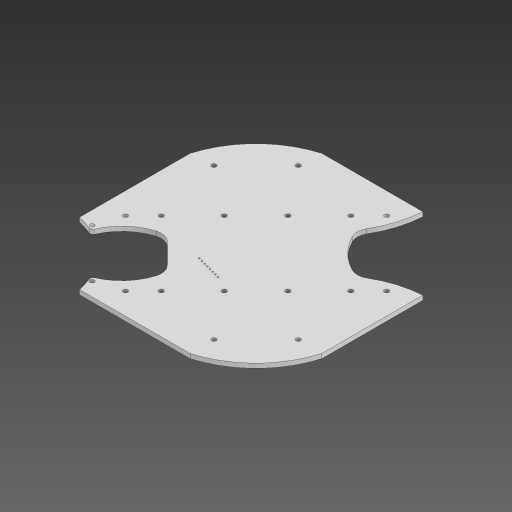
# Autodesk Inventor part: plata_v2
Saved by Autodesk Inventor 2023 (Build 270158000, 158)
## iProperties
Created: 2025-06-24
Part Number: plata_v2
Material: Типовые
Document SubType Name: Modeling
Designer: daa
Density: 1 g/cm^3
Appearance: По умолчанию
Author: daa
Autodesk Inventor part; units mm, degrees
ref_plane "YZ Plane" through (0, 0, 0) normal (1, 0, 0) x (0, 1, 0)
ref_plane "XZ Plane" through (0, 0, 0) normal (0, 1, 0) x (-1, 0, 0)
ref_plane "XY Plane" through (0, 0, 0) normal (0, 0, 1) x (1, 0, 0)
sketch "Эскиз1" plane through (0, 0, 0) normal (0, 1, 0) x (-1, 0, 0)
  line L0 (-79, -47.2724) -> (-79, 14.7276)
  line L1 (91.5447, -47.2724) -> (91.5447, 14.7276)
  line L2 (-79, -47.2724) -> (-93, -47.2724)
  line L3 (-79, 14.7276) -> (-93, 14.7276)
  line L4 (91.5447, -47.2724) -> (105.5447, -47.2724)
  line L5 (91.5447, 14.7276) -> (105.5447, 14.7276)
  line L6 (-24.7276, -101.5447) -> (37.2724, -101.5447)
  line L7 (-24.7276, 69) -> (37.2724, 69)
  line L8 (-24.7276, 69) -> (-24.7276, 83)
  line L9 (37.2724, 69) -> (37.2724, 83)
  line L10 (37.2724, -101.5447) -> (37.2724, -115.5447)
  line L11 (-24.7276, -101.5447) -> (-24.7276, -115.5447)
  arc A0 (-93, -47.2724) -> (-24.7276, -115.5447) centre (6.2724, -16.2724) ccw
  arc A1 (105.5447, 14.7276) -> (37.2724, 83) centre (6.2724, -16.2724) ccw
  arc A2 (-24.7276, 83) -> (-93, 14.7276) centre (6.2724, -16.2724) ccw
  arc A3 (37.2724, -115.5447) -> (105.5447, -47.2724) centre (6.2724, -16.2724) ccw
  dimension "d29" = 62
  dimension "d31" = 62
  dimension "d33" = 14
  dimension "d34" = 14
  dimension "d35" = 62
  dimension "d36" = 62
  dimension "d39" = 14
  dimension "d40" = 14
  constraints: 24 end point, 8 point on circle, 4 centre point, 4 horizontal, 3 parallel, 3 vertical, 2 point on line, 1 concentric
  measures "d29" distance of L0.start L0.end
  measures "d31" distance of L1.start L1.end
  measures "d33" distance of L0.end L3.end
  measures "d34" distance of L1.end L5.end
  measures "d35" distance of L6.start L6.end
  measures "d36" distance of L7.start L7.end
  measures "d39" distance of L7.start L8.end
  measures "d40" distance of L6.start L11.end
extrude "motor" add sketch "Эскиз1" along normal blind 3
sketch "Эскиз2" plane through (0, 3, 0) normal (0, 1, 0) x (1, 0, 0)
  arc A0 (24.7276, -83) -> (93, -14.7276) centre (-6.2724, 16.2724) ccw projected
  arc A1 (-37.2724, 115.5447) -> (-105.5447, 47.2724) centre (-6.2724, 16.2724) ccw projected
  circle A2 centre (-6.2724, 16.2724) radius 104
  line L0 (-6.2724, 16.2724) -> (-6.2724, -50.7276)
  arc A3 (-37.2724, 115.5447) -> (-105.5447, 47.2724) centre (-6.2724, 16.2724) ccw projected
  line L1 (-88.7917, -14.3063) -> (-40.8426, -62.2554)
  line L2 (-101.3809, -25.8032) -> (-48.3479, -78.8362)
  arc A4 (-105.5447, -14.7276) -> (-37.2724, -83) centre (-6.2724, 16.2724) ccw projected
  arc A5 (-48.3479, -78.8362) -> (-101.3809, -25.8032) centre (-98.035, -75.4903) ccw
  arc A6 (24.7276, -83) -> (93, -14.7276) centre (-6.2724, 16.2724) ccw projected
  line L3 (18.2427, 88.7365) -> (66.1918, 40.7874)
  line L4 (34.7276, 111.8495) -> (89.3048, 57.2724)
  arc A7 (34.7276, 111.8495) -> (89.3048, 57.2724) centre (70.9224, 93.4671) ccw
  line L5 (-91.5447, -14.7276) -> (-105.5447, -14.7276) projected
  arc A8 (-105.5447, -14.7276) -> (-101.3809, -25.8032) centre (-6.2724, 16.2724) ccw
  line L6 (-105.5447, -14.7276) -> (-80, -14.7276)
  line L7 (24.7276, 115.5447) -> (24.7276, 101.5447) projected
  line L8 (79, 47.2724) -> (93, 47.2724) projected
  arc A9 (89.3048, 57.2724) -> (34.7276, 111.8495) centre (-6.2724, 16.2724) ccw
  line L9 (93, 47.2724) -> (79, 47.2724)
  line L10 (24.7276, 115.5447) -> (24.7276, 101.5447)
  arc A10 (89.3048, 57.2724) -> (93, 47.2724) centre (-6.2724, 16.2724) ccw
  arc A11 (93, 47.2724) -> (24.7276, 115.5447) centre (-6.2724, 16.2724) ccw projected
  arc A12 (24.7276, 115.5447) -> (34.7276, 111.8495) centre (-6.2724, 16.2724) ccw
  line L11 (79, 47.2724) -> (59.7069, 47.2724)
  line L12 (24.7276, 101.5447) -> (24.7276, 82.2516)
  point P0 (0, 0)
  point P1 (-6.2724, -50.7276)
  point P2 (35.8032, 111.3809)
  point P3 (89.3048, 57.2724)
  point P4 (42.2173, 64.762)
  dimension "d181" = 208
  dimension "d190" = 67
  dimension "d205" = 75
  dimension "d207" = 17.0315
  dimension "d208" = 11.0756
  dimension "d209" = 104
  dimension "d316" = 28
  dimension "d317" = 10
  dimension "d318" = 10
  dimension "d330" = 40.5953
  constraints: 20 end point, 14 point on circle, 7 centre point, 4 point on line, 2 collinear, 2 tangent, 1 horizontal, 1 midpoint, 1 vertical
  measures "d181" diameter of A2
  measures "d190" distance of L0.end L0.start
  measures "d205" distance of L2.start L2.end
  measures "d207" distance between parallel lines of L1 L2
  measures "d208" horizontal distance of A2.end L2.end
  measures "d209" radius of A8
  measures "d316" distance from line of point (42.217, 64.762) L4
  measures "d317" distance from line of L7 L4.start
  measures "d318" distance from line of L4.end L8
  measures "d330" radius of A7
extrude "ball" cut sketch "Эскиз2" against normal blind 3 contours A2 L2 | L2 A5 | L4 A2 | A7 L4
sketch "Эскиз3" plane through (0, 3, 0) normal (0, 1, 0) x (1, 0, 0)
  arc A0 (93, 47.2724) -> (24.7276, 115.5447) centre (-6.2724, 16.2724) ccw projected
  line L0 (-6.2724, 16.2724) -> (97.7276, 16.2724) construction
  line L1 (67.2668, 89.8115) -> (-62.5447, -40)
  circle A1 centre (70.5306, -44.2673) radius 1.5
  circle A2 centre (54.2672, -60.5308) radius 1.5
  circle A3 centre (41.3053, -71.6104) radius 1.5
  circle A4 centre (81.6104, -31.3053) radius 1.5
  arc A5 (24.7276, -83) -> (93, -14.7276) centre (-6.2724, 16.2724) ccw projected
  line L2 (-6.2724, 16.2724) -> (97.7276, 16.2724) construction
  line L3 (-79.8115, 89.8115) -> (67.2668, -57.2668)
  line L4 (-91.5447, 47.2724) -> (-91.5447, -14.7276) projected
  line L5 (-91.5447, 16.2724) -> (79, 16.2724)
  line L6 (24.7276, 101.5447) -> (-37.2724, 101.5447) projected
  line L7 (-6.2724, 101.5447) -> (-6.2724, -69)
  line L8 (-6.2724, 101.5447) -> (-6.2724, -69)
  line L9 (-91.5447, 47.2724) -> (-91.5447, -14.7276) projected
  arc A6 (24.7276, -83) -> (93, -14.7276) centre (-6.2724, 16.2724) ccw projected
  circle A7 centre (-66.812, 93.0753) radius 1.5
  circle A8 centre (-83.0755, 76.8119) radius 1.5
  circle A9 centre (-94.1551, 63.85) radius 1.5
  circle A10 centre (-53.85, 104.1551) radius 1.5
  point P0 (0, 0)
  point P1 (67.2668, -57.2668)
  point P2 (67.2668, -57.2668)
  point P3 (-105.5447, 47.2724)
  point P4 (-79.8115, 89.8115)
  point P5 (-79.8115, 89.8115)
  point P6 (-79.8115, 89.8115)
  dimension "d65" = 3
  dimension "d66" = 3
  dimension "d67" = 3
  dimension "d68" = 3
  dimension "d69" = 23
  dimension "d71" = 57
  dimension "d74" = -12.962
  dimension "d78" = 25.9614
  constraints: 14 end point, 8 centre point, 8 symmetric about line, 4 point on circle, 3 midpoint, 2 horizontal, 2 vertical, 1 point on line, 4 other
  measures "d65" diameter of A1
  measures "d66" diameter of A2
  measures "d67" diameter of A3
  measures "d68" diameter of A4
  measures "d69" distance of A2.centre A1.centre
  measures "d71" distance of A3.centre A4.centre
  measures "d74" vertical distance of A1.centre A4.centre
  measures "d78" vertical distance of A4.centre point (67.267, -57.267)
extrude "hand_mount" cut sketch "Эскиз3" against normal blind 10
sketch "Эскиз5" plane through (0, 3, 0) normal (0, 1, 0) x (1, 0, 0)
  circle A0 centre (29.7645, -47.992) radius 1.5
  circle A1 centre (58.0485, -19.7074) radius 1.5
  circle A2 centre (-6.2982, 16.355) radius 104
  arc A3 (-105.5447, -14.7276) -> (-99.04, -30.7083) centre (-6.2982, 16.355) ccw projected
  line L0 (-6.2982, 16.355) -> (97.7018, 16.355) construction
  circle A4 centre (-71.4195, 53.192) radius 1.5
  circle A5 centre (-43.1349, 81.476) radius 1.5
  circle A6 centre (-45.0925, -54.9329) radius 1.5
  line L1 (-62.8214, -40.2767) -> (-61.356, -38.6694)
  line L2 (-61.356, -38.6694) -> (-45.4214, -38.6694) construction
  circle A7 centre (-77.6194, -22.406) radius 1.5
  arc A8 (24.7276, -83) -> (93, -14.7276) centre (-6.2724, 16.2724) ccw projected
  line L3 (-6.2982, 16.355) -> (97.7785, 16.355) construction
  line L4 (64.1086, -60.2947) -> (-82.2655, 87.2726)
  arc A9 (-37.2724, 115.5447) -> (-105.5447, 47.2724) centre (-6.2724, 16.2724) ccw projected
  circle A10 centre (27.3717, 81.7363) radius 1.5
  arc A11 (-48.3479, -78.8362) -> (-101.3809, -25.8032) centre (-98.035, -75.4903) ccw projected
  arc A12 (34.7276, 111.8495) -> (89.3048, 57.2724) centre (70.9224, 93.4671) ccw projected
  circle A13 centre (59.1841, 49.909) radius 1.5
  line L5 (27.3717, 81.7363) -> (71.0459, 81.7363) construction
  line L6 (27.3717, 81.7363) -> (59.1841, 49.909)
  line L7 (42.2173, 64.762) -> (43.2779, 65.8226)
  line L8 (42.2173, 64.762) -> (43.7173, 64.762) construction
  line L9 (-77.6194, -22.406) -> (-45.0925, -54.9329)
  line L10 (-77.6194, -22.406) -> (-31.6194, -22.406) construction
  point P0 (0, 0)
  point P1 (-62.8214, -40.2767)
  dimension "d116" = 3
  dimension "d117" = 3
  dimension "d118" = 40
  dimension "d119" = 208
  dimension "d121" = 64.347
  dimension "d126" = 3
  dimension "d130" = 2.175
  dimension "d332" = 45
  dimension "d335" = 1.5
  dimension "d336" = 45
  dimension "d337" = 46
  dimension "d338" = 45
  constraints: 22 end point, 9 centre point, 6 horizontal, 5 point on circle, 2 equal length, 2 midpoint, 1 coincident, 1 concentric, 1 symmetric about line, 1 other
  measures "d116" diameter of A0
  measures "d117" diameter of A1
  measures "d118" distance of A1.centre A0.centre
  measures "d119" diameter of A2
  measures "d121" vertical distance of L0.start A0.centre
  measures "d126" diameter of A6
  measures "d130" distance of L1.end L1.start
  measures "d332" distance of L5.start L6.end
  measures "d335" distance of L7.end L7.start
  measures "d336" angle of L8 L7
  measures "d337" distance of L9.start L9.end
  measures "d338" angle of L9 L10
extrude "Выдавливание5" cut sketch "Эскиз5" against normal blind 10 contours A0 | A1 | A4 | A5 | A6 | A7 | A10 | A13
sketch "Эскиз9" plane through (0, 3, 0) normal (0, 1, 0) x (1, 0, 0)
  line L0 (-38.87, 27.5154) -> (-17.5154, 48.87)
  line L1 (-17.5154, 48.87) -> (26.3253, 5.0294)
  line L2 (26.3253, 5.0294) -> (4.9706, -16.3253)
  line L3 (4.9706, -16.3253) -> (-38.87, 27.5154)
  circle A0 centre (-6.2724, 16.2724) radius 104
  arc A1 (-37.2724, 115.5447) -> (-105.5447, 47.2724) centre (-6.2724, 16.2724) ccw projected
  circle A2 centre (-17.5154, 48.87) radius 1.5
  circle A3 centre (-38.87, 27.5154) radius 1.5
  circle A4 centre (4.9706, -16.3253) radius 1.5
  circle A5 centre (26.3253, 5.0294) radius 1.5
  point P0 (0, 0)
  point P1 (-39.9194, 114.679)
  point P2 (-104.679, 49.9194)
  dimension "d224" = 30.2
  dimension "d225" = 62
  dimension "d226" = 208
  dimension "d227" = 15.1
  dimension "d229" = 31
  dimension "d230" = 3
  dimension "d231" = 3
  dimension "d232" = 3
  dimension "d233" = 3
  constraints: 8 end point, 5 centre point, 4 coincident, 2 parallel, 1 concentric, 1 perpendicular
  measures "d224" distance of L1.end L2.end
  measures "d225" distance of L0.end L1.end
  measures "d226" diameter of A0
  measures "d227" distance from line of L1 A0.centre
  measures "d229" distance from line of L2 A0.centre
  measures "d230" diameter of A2
  measures "d231" diameter of A3
  measures "d232" diameter of A4
  measures "d233" diameter of A5
extrude "Выдавливание8" cut sketch "Эскиз9" against normal blind 10 contours L3 A3 L0 | L0 A3 L3 | A2 L1 L0 | L0 L1 A2 | A4 L2 L3 | L3 L2 A4 | A5 L2 L1 | L1 L2 A5
sketch "Эскиз8" plane through (0, 3, 0) normal (0, 1, 0) x (1, 0, 0)
  circle A0 centre (62.3989, -52.3991) radius 1.6
  circle A1 centre (54.2672, -60.5308) radius 1.5
  circle A2 centre (54.2672, -60.5308) radius 1.5 projected
  line L0 (54.2672, -60.5308) -> (67.7672, -60.5308) construction
  circle A3 centre (70.5306, -44.2673) radius 1.5
  circle A4 centre (70.5306, -44.2673) radius 1.5 projected
  line L1 (70.5306, -44.2673) -> (82.0306, -44.2673) construction
  line L2 (70.5306, -44.2673) -> (60.52, -44.2673)
  circle A5 centre (70.5306, -44.2673) radius 1.5 projected
  line L3 (60.52, -44.2673) -> (70.5306, -44.2673)
  line L4 (70.5306, -44.2673) -> (62.3989, -52.3991)
  arc A6 (34.7276, 111.8495) -> (89.3048, 57.2724) centre (70.9224, 93.4671) ccw projected
  arc A7 (93, 47.2724) -> (89.3048, 57.2724) centre (-6.2724, 16.2724) ccw projected
  line L5 (24.7276, 115.5447) -> (24.7276, 101.5447) projected
  line L6 (24.7276, 101.5447) -> (-37.2724, 101.5447) projected
  line L7 (-37.2724, 101.5447) -> (-37.2724, 115.5447) projected
  arc A8 (-37.2724, 115.5447) -> (-105.5447, 47.2724) centre (-6.2724, 16.2724) ccw projected
  line L8 (-105.5447, 47.2724) -> (-91.5447, 47.2724) projected
  line L9 (-91.5447, 47.2724) -> (-91.5447, -14.7276) projected
  line L10 (-91.5447, -14.7276) -> (-105.5447, -14.7276) projected
  arc A9 (-105.5447, -14.7276) -> (-101.3809, -25.8032) centre (-6.2724, 16.2724) ccw projected
  arc A10 (-48.3479, -78.8362) -> (-101.3809, -25.8032) centre (-98.035, -75.4903) ccw projected
  arc A11 (-48.3479, -78.8362) -> (-37.2724, -83) centre (-6.2724, 16.2724) ccw projected
  line L11 (-37.2724, -83) -> (-37.2724, -69) projected
  line L12 (-37.2724, -69) -> (24.7276, -69) projected
  line L13 (24.7276, -69) -> (24.7276, -83) projected
  arc A12 (24.7276, -83) -> (93, -14.7276) centre (-6.2724, 16.2724) ccw projected
  line L14 (93, -14.7276) -> (79, -14.7276) projected
  line L15 (79, -14.7276) -> (79, 47.2724) projected
  line L16 (79, 47.2724) -> (93, 47.2724) projected
  arc A13 (34.7276, 111.8495) -> (24.7276, 115.5447) centre (-6.2724, 16.2724) ccw projected
  circle A14 centre (-94.1551, 63.85) radius 1.5 projected
  circle A15 centre (41.3053, -71.6104) radius 1.5 projected
  circle A16 centre (81.6104, -31.3053) radius 1.5 projected
  circle A17 centre (-53.85, 104.1551) radius 1.5 projected
  circle A18 centre (-83.0755, 76.8119) radius 1.5 projected
  circle A19 centre (54.2672, -60.5308) radius 1.5 projected
  circle A20 centre (70.5306, -44.2673) radius 1.5 projected
  circle A21 centre (-66.812, 93.0753) radius 1.5 projected
  circle A22 centre (-45.0925, -54.9329) radius 1.5 projected
  circle A23 centre (29.7645, -47.992) radius 1.5 projected
  circle A24 centre (-43.1349, 81.476) radius 1.5 projected
  circle A25 centre (27.3717, 81.7363) radius 1.5 projected
  circle A26 centre (-77.6194, -22.406) radius 1.5 projected
  circle A27 centre (58.0485, -19.7074) radius 1.5 projected
  circle A28 centre (-71.4195, 53.192) radius 1.5 projected
  line L17 (42.2173, 64.762) -> (-62.8214, -40.2767)
  arc A29 (-48.275, -77.4757) -> (-100.0204, -25.7303) centre (-98.035, -75.4903) ccw projected
  circle A30 centre (-74.9438, 84.9436) radius 1.6
  point P0 (0, 0)
  dimension "d212" = 3.2
  dimension "d216" = 3
  dimension "d221" = 3
  dimension "d311" = 11.5
  dimension "d312" = 45
  constraints: 12 end point, 4 centre point, 3 horizontal, 3 point on circle, 2 concentric, 1 coincident, 1 collinear, 1 symmetric about line, 1 other
  measures "d212" diameter of A0
  measures "d216" diameter of A1
  measures "d221" diameter of A3
  measures "d311" distance of L3.end L4.end
  measures "d312" angle of L3 L4
extrude "Выдавливание7" cut sketch "Эскиз8" against normal blind 10 contours A0 | A30
sketch "Эскиз10" plane through (0, 3, 0) normal (0, 1, 0) x (1, 0, 0)
  circle A0 centre (-6.2724, 16.2719) radius 104.0005
  arc A1 (-37.2724, 115.5447) -> (-105.5447, 47.2724) centre (-6.2724, 16.2724) ccw projected
  line L0 (-60.0125, 6.3729) -> (-72.0333, -5.648)
  line L1 (-72.0333, -5.648) -> (-28.1927, -49.4886)
  line L2 (-28.1927, -49.4886) -> (-16.1718, -37.4678)
  line L3 (-16.1718, -37.4678) -> (-60.0125, 6.3729)
  circle A2 centre (-60.0125, 6.3729) radius 1.5
  circle A3 centre (-72.0333, -5.648) radius 1.5
  circle A4 centre (-16.1718, -37.4678) radius 1.5
  circle A5 centre (-28.1927, -49.4886) radius 1.5
  arc A6 (24.7276, -83) -> (93, -14.7276) centre (-6.2724, 16.2724) ccw projected
  line L4 (-6.2724, 16.2724) -> (97.7276, 16.2724) construction
  line L5 (67.2668, -57.2668) -> (-79.8115, 89.8115)
  line L6 (3.6271, 70.0125) -> (15.648, 82.0333)
  line L7 (15.648, 82.0333) -> (59.4886, 38.1927)
  line L8 (59.4886, 38.1927) -> (47.4678, 26.1718)
  line L9 (47.4678, 26.1718) -> (3.6271, 70.0125)
  circle A7 centre (3.6271, 70.0125) radius 1.5
  circle A8 centre (15.648, 82.0333) radius 1.5
  circle A9 centre (47.4678, 26.1718) radius 1.5
  circle A10 centre (59.4886, 38.1927) radius 1.5
  point P0 (0, 0)
  point P1 (-39.9194, 114.679)
  point P2 (-104.679, 49.9194)
  point P3 (27.3747, -82.1343)
  point P4 (92.1343, -17.3747)
  point P5 (10, 10)
  point P6 (-6.2719, 16.2724)
  dimension "d248" = 17
  dimension "d249" = 62
  dimension "d250" = 9.899
  dimension "d251" = 45
  dimension "d252" = 3
  dimension "d253" = 3
  dimension "d254" = 3
  dimension "d255" = 3
  constraints: 20 end point, 10 symmetric about line, 9 centre point, 8 coincident, 2 parallel, 2 point on circle, 1 horizontal, 1 perpendicular, 1 tangent, 4 other
  measures "d248" distance of L2.end L1.end
  measures "d249" distance of L1.end L0.end
  measures "d250" vertical distance of L0.start A0.centre
  measures "d251" distance from line of L3 L4.start
  measures "d252" diameter of A2
  measures "d253" diameter of A3
  measures "d254" diameter of A4
  measures "d255" diameter of A5
extrude "Выдавливание9" cut sketch "Эскиз10" against normal blind 10 contours L3 A2 L0 | L0 A2 L3 | A3 L1 L0 | L0 L1 A3 | A4 L2 L3 | L3 L2 A4 | A5 L2 L1 | L1 L2 A5 | L9 A7 L6 | L6 A7 L9 | A8 L7 L6 | L6 L7 A8 | A9 L8 L9 | L9 L8 A9 | A10 L8 L7 | L7 L8 A10
sketch "Эскиз19" plane through (0, 3, 0) normal (0, 1, 0) x (1, 0, 0)
  circle A0 centre (47.4678, 26.1718) radius 1.5 projected
  circle A1 centre (-28.1927, -49.4886) radius 1.5 projected
  circle A2 centre (-72.0333, -5.648) radius 1.5 projected
  circle A3 centre (15.648, 82.0333) radius 1.5 projected
  circle A4 centre (59.4886, 38.1927) radius 1.5 projected
  circle A5 centre (-16.1718, -37.4678) radius 1.5 projected
  circle A6 centre (-60.0125, 6.3729) radius 1.5 projected
  circle A7 centre (3.6271, 70.0125) radius 1.5 projected
  circle A8 centre (4.9706, -16.3253) radius 1.5 projected
  circle A9 centre (-17.5154, 48.87) radius 1.5 projected
  circle A10 centre (26.3253, 5.0294) radius 1.5 projected
  circle A11 centre (-38.87, 27.5154) radius 1.5 projected
  circle A12 centre (62.3989, -52.3991) radius 1.6 projected
  circle A13 centre (-74.9438, 84.9436) radius 1.6 projected
  circle A14 centre (58.0485, -19.7074) radius 1.5 projected
  circle A15 centre (-71.4195, 53.192) radius 1.5 projected
  circle A16 centre (27.3717, 81.7363) radius 1.5 projected
  circle A17 centre (-77.6194, -22.406) radius 1.5 projected
  circle A18 centre (29.7645, -47.992) radius 1.5 projected
  circle A19 centre (-43.1349, 81.476) radius 1.5 projected
  circle A20 centre (59.1841, 49.909) radius 1.5 projected
  circle A21 centre (-45.0925, -54.9329) radius 1.5 projected
  circle A22 centre (-66.812, 93.0753) radius 1.5 projected
  circle A23 centre (70.5306, -44.2673) radius 1.5 projected
  circle A24 centre (54.2672, -60.5308) radius 1.5 projected
  circle A25 centre (-83.0755, 76.8119) radius 1.5 projected
  circle A26 centre (-53.85, 104.1551) radius 1.5 projected
  circle A27 centre (81.6104, -31.3053) radius 1.5 projected
  circle A28 centre (41.3053, -71.6104) radius 1.5 projected
  circle A29 centre (-94.1551, 63.85) radius 1.5 projected
  arc A30 (34.7276, 111.8495) -> (89.3048, 57.2724) centre (70.9224, 93.4671) ccw projected
  arc A31 (34.7276, 111.8495) -> (24.7276, 115.5447) centre (-6.2724, 16.2724) ccw projected
  line L0 (24.7276, 115.5447) -> (24.7276, 101.5447) projected
  line L1 (24.7276, 101.5447) -> (-37.2724, 101.5447) projected
  line L2 (-37.2724, 101.5447) -> (-37.2724, 115.5447) projected
  arc A32 (-37.2724, 115.5447) -> (-105.5447, 47.2724) centre (-6.2724, 16.2724) ccw projected
  line L3 (-105.5447, 47.2724) -> (-91.5447, 47.2724) projected
  line L4 (-91.5447, 47.2724) -> (-91.5447, -14.7276) projected
  line L5 (-91.5447, -14.7276) -> (-105.5447, -14.7276) projected
  arc A33 (-105.5447, -14.7276) -> (-101.3809, -25.8032) centre (-6.2724, 16.2724) ccw projected
  arc A34 (-48.3479, -78.8362) -> (-101.3809, -25.8032) centre (-98.035, -75.4903) ccw projected
  arc A35 (-48.3479, -78.8362) -> (-37.2724, -83) centre (-6.2724, 16.2724) ccw projected
  line L6 (-37.2724, -83) -> (-37.2724, -69) projected
  line L7 (-37.2724, -69) -> (24.7276, -69) projected
  line L8 (24.7276, -69) -> (24.7276, -83) projected
  arc A36 (24.7276, -83) -> (93, -14.7276) centre (-6.2724, 16.2724) ccw projected
  line L9 (93, -14.7276) -> (79, -14.7276) projected
  line L10 (79, -14.7276) -> (79, 47.2724) projected
  line L11 (79, 47.2724) -> (93, 47.2724) projected
  arc A37 (93, 47.2724) -> (89.3048, 57.2724) centre (-6.2724, 16.2724) ccw projected
  arc A38 (-42.2724, 108.4949) -> (-98.4949, 52.2724) centre (-6.2724, 16.2724) ccw
  line L12 (-42.2724, 108.4949) -> (-42.2724, 96.5447)
  line L13 (-42.2724, 96.5447) -> (25.4312, 96.5447)
  arc A39 (25.4312, 96.5447) -> (74, 47.9759) centre (70.9224, 93.4671) ccw
  line L14 (74, 47.9759) -> (74, -19.7276)
  line L15 (74, -19.7276) -> (85.9502, -19.7276)
  arc A40 (29.7276, -75.9502) -> (85.9502, -19.7276) centre (-6.2724, 16.2724) ccw
  line L16 (29.7276, -75.9502) -> (29.7276, -64)
  line L17 (-86.5447, 52.2724) -> (-98.4949, 52.2724)
  arc A41 (-42.2724, 96.5447) -> (-86.5447, 52.2724) centre (-24.1284, 34.1284) ccw
  arc A42 (29.7276, -64) -> (74, -19.7276) centre (11.5837, -1.5837) ccw
  line L18 (-86.5447, 52.2724) -> (-86.5447, -21.9089)
  line L19 (29.7276, -64) -> (-44.4536, -64)
  arc A43 (-44.4536, -64) -> (-86.5447, -21.9089) centre (-98.035, -75.4903) ccw
  point P0 (0, 0)
  point P1 (26.5474, 82.9894)
  point P2 (27.2884, 80.2386)
  point P3 (57.6859, 49.8355)
  point P4 (60.4425, 49.0926)
  dimension "d339" = 5
  dimension "d340" = 65
  dimension "d341" = 65
  constraints: 16 end point, 12 point on circle, 6 centre point, 1 perpendicular, 1 vertical, 7 other
  measures "d339" radial gap between concentric circles of A32 A38
  measures "d340" radius of A41
  measures "d341" radius of A42
extrude "Выдавливание13" cut sketch "Эскиз19" against normal blind 10 contours A41 L17 A38 A29 A25 A22 A26 L12 | L15 A40 A27 A23 A24 A28 L16 A42 | A30 A37 L11 L10 L9 A36 L8 L7 L6 A35 A34 A33 L5 L4 L3 A32 L2 L1 L0 A31
sketch "Эскиз20" plane through (0, 3, 0) normal (0, 1, 0) x (1, 0, 0)
  circle A0 centre (-45.0925, -54.9329) radius 1.5 projected
  circle A1 centre (-43.1349, 81.476) radius 1.5 projected
  circle A2 centre (29.7645, -47.992) radius 1.5 projected
  circle A3 centre (-77.6194, -22.406) radius 1.5 projected
  circle A4 centre (-71.4195, 53.192) radius 1.5 projected
  circle A5 centre (58.0485, -19.7074) radius 1.5 projected
  circle A6 centre (-38.87, 27.5154) radius 1.5 projected
  circle A7 centre (26.3253, 5.0294) radius 1.5 projected
  circle A8 centre (-17.5154, 48.87) radius 1.5 projected
  circle A9 centre (4.9706, -16.3253) radius 1.5 projected
  circle A10 centre (3.6271, 70.0125) radius 1.5 projected
  circle A11 centre (-60.0125, 6.3729) radius 1.5 projected
  circle A12 centre (-16.1718, -37.4678) radius 1.5 projected
  circle A13 centre (59.4886, 38.1927) radius 1.5 projected
  circle A14 centre (15.648, 82.0333) radius 1.5 projected
  circle A15 centre (-72.0333, -5.648) radius 1.5 projected
  circle A16 centre (-28.1927, -49.4886) radius 1.5 projected
  circle A17 centre (47.4678, 26.1718) radius 1.5 projected
  arc A18 (25.4312, 96.5447) -> (26.5474, 82.9894) centre (70.9224, 93.4671) ccw projected
  line L0 (25.4312, 96.5447) -> (-42.2724, 96.5447) projected
  arc A19 (-42.2724, 96.5447) -> (-86.5447, 52.2724) centre (-24.1284, 34.1284) ccw projected
  line L1 (-86.5447, 52.2724) -> (-86.5447, -21.9089) projected
  arc A20 (-44.4536, -64) -> (-86.5447, -21.9089) centre (-98.035, -75.4903) ccw projected
  line L2 (-44.4536, -64) -> (29.7276, -64) projected
  arc A21 (29.7276, -64) -> (74, -19.7276) centre (11.5837, -1.5837) ccw projected
  line L3 (74, -19.7276) -> (74, 47.9759) projected
  arc A22 (60.4425, 49.0926) -> (74, 47.9759) centre (70.9224, 93.4671) ccw projected
  arc A23 (57.6859, 49.8355) -> (60.4425, 49.0926) centre (59.1841, 49.909) ccw projected
  arc A24 (27.2884, 80.2386) -> (57.6859, 49.8355) centre (70.9224, 93.4671) ccw projected
  arc A25 (26.5474, 82.9894) -> (27.2884, 80.2386) centre (27.3717, 81.7363) ccw projected
  arc A26 (-44.4536, -64) -> (-86.5447, -21.9089) centre (-98.035, -75.4903) ccw projected
  line L4 (-71.3723, -27.6144) -> (-50.1591, -48.8276)
  line L5 (-50.1591, -48.8276) -> (-25.4104, -24.0789)
  line L6 (-25.4104, -24.0789) -> (-46.6236, -2.8657)
  line L7 (-46.6236, -2.8657) -> (-71.3723, -27.6144)
  arc A27 (-46.6236, -2.8657) -> (-75.3457, -25.6085) centre (-42.4708, -37.6184) ccw
  line L8 (-36.017, -13.4723) -> (-60.7657, -38.221)
  arc A28 (-48.1532, -52.801) -> (-25.4104, -24.0789) centre (-60.1632, -19.9261) ccw
  line L9 (-8.4206, 14.1241) -> (55.3471, -49.6436)
  arc A29 (29.7276, -64) -> (74, -19.7276) centre (11.5837, -1.5837) ccw projected
  line L10 (-8.4206, 14.1241) -> (81.7606, 14.1241) construction
  line L11 (55.3471, -49.6436) -> (-72.1883, 77.8919)
  arc A30 (-42.2724, 96.5447) -> (-86.5447, 52.2724) centre (-24.1284, 34.1284) ccw projected
  line L12 (28.0624, 77.9125) -> (55.3265, 50.6222)
  line L13 (55.3265, 50.6222) -> (41.1775, 36.4868)
  line L14 (41.1775, 36.4868) -> (13.9134, 63.7772)
  line L15 (13.9134, 63.7772) -> (28.0624, 77.9125)
  arc A31 (26.5474, 82.9894) -> (27.2884, 80.2386) centre (27.3717, 81.7363) ccw projected
  arc A32 (13.9134, 63.7772) -> (41.1775, 36.4868) centre (56.3081, 78.8669) ccw
  arc A33 (13.9134, 63.7772) -> (25.4312, 96.5447) centre (-39.4206, 100.932) ccw
  arc A34 (74, 47.9759) -> (41.1775, 36.4868) centre (78.2808, -16.883) ccw
  point P0 (0, 0)
  point P1 (-75.3457, -25.6085)
  point P2 (73.9122, 47.97)
  dimension "d357" = 35
  dimension "d363" = 35
  dimension "d368" = 45
  dimension "d369" = 20
  dimension "d372" = 45
  dimension "d382" = 65
  dimension "d383" = 65
  constraints: 24 end point, 17 point on circle, 5 centre point, 4 parallel, 2 midpoint, 2 perpendicular, 2 symmetric about line, 1 equal length, 1 horizontal, 1 point on line, 1 tangent, 1 other
  measures "d357" distance of L5.end L4.end
  measures "d363" radius of A27
  measures "d368" angle of L9 L10
  measures "d369" distance of L12.end L13.end
  measures "d372" radius of A32
  measures "d382" radius of A33
  measures "d383" radius of A34
extrude "Выдавливание14" cut sketch "Эскиз20" against normal blind 10 contours A18 A25 A24 L15 A33 | L15 A24 L13 L14 | L14 A32 | L13 A24 A23 A22 A34 | A27 L7 A20 | L7 L6 L8 A20 | L8 L6 L5 A20 | A20 L5 A28
fillet "Сопряжение12" radius 10 2 edges at (-46.6236, 1.5, 2.8657) (-25.4104, 1.5, 24.0789)
fillet "Сопряжение13" radius 2 2 edges at (-75.3457, 1.5, 25.6085) (-48.1532, 1.5, 52.801)
fillet "Сопряжение14" radius 10 2 edges at (13.9134, 1.5, -63.7772) (41.1775, 1.5, -36.4868)
sketch "Эскиз21" plane through (0, 3, 0) normal (0, 1, 0) x (1, 0, 0)
  circle A0 centre (9.8791, 38.23) radius 0.45 projected
  circle A1 centre (7.4254, 38.8877) radius 0.45 projected
  circle A2 centre (4.9725, 39.5446) radius 0.45 projected
  ellipse E0 centre (-6.272, 16.272) end of major axis (-21.0463, 59.1087) minor radius 45.313 projected
  circle A3 centre (-12.1713, -26.3968) radius 0.425 projected
  circle A4 centre (-17.1529, -25.4059) radius 0.425 projected
  circle A5 centre (-14.6618, -25.9017) radius 0.425 projected
  circle A6 centre (-3.7334, -26.7287) radius 0.425 projected
  circle A7 centre (-8.8133, -26.7285) radius 0.425 projected
  circle A8 centre (-6.2734, -26.7286) radius 0.425 projected
  circle A9 centre (-30.1627, -19.4807) radius 0.425 projected
  circle A10 centre (-34.8635, -15.9096) radius 0.425 projected
  circle A11 centre (-32.2833, -18.0827) radius 0.425 projected
  circle A12 centre (-22.7291, -23.4541) radius 0.425 projected
  circle A13 centre (-20.3822, -24.4265) radius 0.425 projected
  circle A14 centre (-28.0422, -20.8787) radius 0.425 projected
  circle A15 centre (-25.0752, -22.4825) radius 0.425 projected
  circle A16 centre (17.6165, -19.4822) radius 0.425 projected
  circle A17 centre (12.5287, -22.4837) radius 0.425 projected
  circle A18 centre (15.5043, -20.8928) radius 0.425 projected
  circle A19 centre (24.1326, -14.1346) radius 0.425 projected
  circle A20 centre (25.9287, -12.3386) radius 0.425 projected
  circle A21 centre (19.7279, -18.0709) radius 0.425 projected
  circle A22 centre (22.3365, -15.9306) radius 0.425 projected
  circle A23 centre (4.6062, -25.4066) radius 0.425 projected
  circle A24 centre (-0.3754, -26.3971) radius 0.425 projected
  circle A25 centre (2.1151, -25.9022) radius 0.425 projected
  circle A26 centre (7.8356, -24.4274) radius 0.425 projected
  circle A27 centre (10.1825, -23.4552) radius 0.425 projected
  ellipse E1 centre (4.9707, -16.3253) end of major axis (3.8747, -15.2292) minor radius 1.55 projected
  line L0 (19.1105, -0.9108) -> (18.6169, -1.4765) projected
  line L1 (18.6169, -1.4765) -> (11.4756, -8.6187) projected
  line L2 (11.4756, -8.6187) -> (10.9099, -9.1123) projected
  line L3 (10.9099, -9.1123) -> (10.282, -9.5238) projected
  line L4 (10.282, -9.5238) -> (9.6046, -9.8462) projected
  line L5 (9.6046, -9.8462) -> (8.8882, -10.0732) projected
  line L6 (8.8882, -10.0732) -> (8.1486, -10.2004) projected
  line L7 (8.1486, -10.2004) -> (7.3984, -10.2266) projected
  line L8 (7.3984, -10.2266) -> (6.6524, -10.1495) projected
  line L9 (6.6524, -10.1495) -> (5.9226, -9.9713) projected
  line L10 (5.9226, -9.9713) -> (5.2247, -9.6962) projected
  line L11 (5.2247, -9.6962) -> (4.57, -9.3285) projected
  line L12 (4.57, -9.3285) -> (3.9718, -8.8745) projected
  line L13 (3.9718, -8.8745) -> (3.4415, -8.3441) projected
  line L14 (3.4415, -8.3441) -> (2.9875, -7.7459) projected
  line L15 (2.9875, -7.7459) -> (2.6198, -7.0911) projected
  line L16 (2.6198, -7.0911) -> (2.3448, -6.3932) projected
  line L17 (2.3448, -6.3932) -> (2.1666, -5.6634) projected
  line L18 (2.1666, -5.6634) -> (2.0896, -4.9174) projected
  line L19 (2.0896, -4.9174) -> (2.1158, -4.1672) projected
  line L20 (2.1158, -4.1672) -> (2.2431, -3.4276) projected
  line L21 (2.2431, -3.4276) -> (2.4701, -2.7113) projected
  line L22 (2.4701, -2.7113) -> (2.7925, -2.0339) projected
  line L23 (2.7925, -2.0339) -> (3.2041, -1.406) projected
  line L24 (3.2041, -1.406) -> (3.6977, -0.8403) projected
  line L25 (3.6977, -0.8403) -> (10.839, 6.3019) projected
  line L26 (10.839, 6.3019) -> (11.4047, 6.7955) projected
  line L27 (11.4047, 6.7955) -> (12.0326, 7.207) projected
  line L28 (12.0326, 7.207) -> (12.71, 7.5294) projected
  line L29 (12.71, 7.5294) -> (13.4263, 7.7564) projected
  line L30 (13.4263, 7.7564) -> (14.166, 7.8836) projected
  line L31 (14.166, 7.8836) -> (14.9162, 7.9098) projected
  line L32 (14.9162, 7.9098) -> (15.6622, 7.8327) projected
  line L33 (15.6622, 7.8327) -> (16.3919, 7.6545) projected
  line L34 (16.3919, 7.6545) -> (17.0898, 7.3794) projected
  line L35 (17.0898, 7.3794) -> (17.7446, 7.0117) projected
  line L36 (17.7446, 7.0117) -> (18.3428, 6.5577) projected
  line L37 (18.3428, 6.5577) -> (18.8731, 6.0273) projected
  line L38 (18.8731, 6.0273) -> (19.3271, 5.4291) projected
  line L39 (19.3271, 5.4291) -> (19.6947, 4.7743) projected
  line L40 (19.6947, 4.7743) -> (19.9698, 4.0764) projected
  line L41 (19.9698, 4.0764) -> (20.1479, 3.3466) projected
  line L42 (20.1479, 3.3466) -> (20.225, 2.6006) projected
  line L43 (20.225, 2.6006) -> (20.1988, 1.8504) projected
  line L44 (20.1988, 1.8504) -> (20.0715, 1.1108) projected
  line L45 (20.0715, 1.1108) -> (19.8445, 0.3945) projected
  line L46 (19.8445, 0.3945) -> (19.522, -0.2829) projected
  line L47 (19.522, -0.2829) -> (19.1105, -0.9108) projected
  circle A28 centre (-36.6786, -14.1326) radius 0.425 projected
  circle A29 centre (-38.4936, -12.3556) radius 0.425 projected
  circle A30 centre (-40.5689, -9.6975) radius 0.425 projected
  circle A31 centre (-42.0262, -7.6164) radius 0.425 projected
  circle A32 centre (-43.4828, -5.5361) radius 0.425 projected
  circle A33 centre (-45.0475, -2.5372) radius 0.425 projected
  circle A34 centre (-45.9992, -0.1825) radius 0.425 projected
  circle A35 centre (-46.9502, 2.1729) radius 0.425 projected
  circle A36 centre (-47.9506, 5.3938) radius 0.425 projected
  circle A37 centre (-48.4462, 7.885) radius 0.425 projected
  circle A38 centre (-48.9411, 10.3754) radius 0.425 projected
  circle A39 centre (-49.2726, 13.7335) radius 0.425 projected
  circle A40 centre (-49.2726, 16.2734) radius 0.425 projected
  circle A41 centre (-49.2725, 18.8133) radius 0.425 projected
  circle A42 centre (-48.8863, 22.1607) radius 0.425 projected
  circle A43 centre (-48.4457, 24.6618) radius 0.425 projected
  circle A44 centre (-48.0044, 27.1635) radius 0.425 projected
  ellipse E2 centre (-38.8699, 27.5153) end of major axis (-39.9659, 28.6114) minor radius 1.55 projected
  line L48 (-15.3379, 34.5779) -> (-15.7495, 33.95) projected
  line L49 (-15.7495, 33.95) -> (-16.243, 33.3843) projected
  line L50 (-16.243, 33.3843) -> (-23.3843, 26.242) projected
  line L51 (-23.3843, 26.242) -> (-23.95, 25.7485) projected
  line L52 (-23.95, 25.7485) -> (-24.578, 25.337) projected
  line L53 (-24.578, 25.337) -> (-25.2554, 25.0146) projected
  line L54 (-25.2554, 25.0146) -> (-25.9717, 24.7876) projected
  line L55 (-25.9717, 24.7876) -> (-26.7113, 24.6604) projected
  line L56 (-26.7113, 24.6604) -> (-27.4616, 24.6342) projected
  line L57 (-27.4616, 24.6342) -> (-28.2076, 24.7113) projected
  line L58 (-28.2076, 24.7113) -> (-28.9373, 24.8895) projected
  line L59 (-28.9373, 24.8895) -> (-29.6352, 25.1646) projected
  line L60 (-29.6352, 25.1646) -> (-30.29, 25.5323) projected
  line L61 (-30.29, 25.5323) -> (-30.8882, 25.9863) projected
  line L62 (-30.8882, 25.9863) -> (-31.4185, 26.5167) projected
  line L63 (-31.4185, 26.5167) -> (-31.8724, 27.1149) projected
  line L64 (-31.8724, 27.1149) -> (-32.2401, 27.7697) projected
  line L65 (-32.2401, 27.7697) -> (-32.5151, 28.4676) projected
  line L66 (-32.5151, 28.4676) -> (-32.6933, 29.1973) projected
  line L67 (-32.6933, 29.1973) -> (-32.7704, 29.9433) projected
  line L68 (-32.7704, 29.9433) -> (-32.7442, 30.6936) projected
  line L69 (-32.7442, 30.6936) -> (-32.6169, 31.4332) projected
  line L70 (-32.6169, 31.4332) -> (-32.3899, 32.1495) projected
  line L71 (-32.3899, 32.1495) -> (-32.0674, 32.8269) projected
  line L72 (-32.0674, 32.8269) -> (-31.6558, 33.4548) projected
  line L73 (-31.6558, 33.4548) -> (-31.1623, 34.0205) projected
  line L74 (-31.1623, 34.0205) -> (-24.021, 41.1627) projected
  line L75 (-24.021, 41.1627) -> (-23.4553, 41.6563) projected
  line L76 (-23.4553, 41.6563) -> (-22.8273, 42.0678) projected
  line L77 (-22.8273, 42.0678) -> (-22.1499, 42.3902) projected
  line L78 (-22.1499, 42.3902) -> (-21.4336, 42.6172) projected
  line L79 (-21.4336, 42.6172) -> (-20.694, 42.7444) projected
  line L80 (-20.694, 42.7444) -> (-19.9437, 42.7706) projected
  line L81 (-19.9437, 42.7706) -> (-19.1977, 42.6935) projected
  line L82 (-19.1977, 42.6935) -> (-18.468, 42.5152) projected
  line L83 (-18.468, 42.5152) -> (-17.7701, 42.2402) projected
  line L84 (-17.7701, 42.2402) -> (-17.1153, 41.8724) projected
  line L85 (-17.1153, 41.8724) -> (-16.5171, 41.4185) projected
  line L86 (-16.5171, 41.4185) -> (-15.9868, 40.8881) projected
  line L87 (-15.9868, 40.8881) -> (-15.5329, 40.2899) projected
  line L88 (-15.5329, 40.2899) -> (-15.1652, 39.6351) projected
  line L89 (-15.1652, 39.6351) -> (-14.8902, 38.9372) projected
  line L90 (-14.8902, 38.9372) -> (-14.712, 38.2074) projected
  line L91 (-14.712, 38.2074) -> (-14.6349, 37.4614) projected
  line L92 (-14.6349, 37.4614) -> (-14.6611, 36.7112) projected
  line L93 (-14.6611, 36.7112) -> (-14.7884, 35.9716) projected
  line L94 (-14.7884, 35.9716) -> (-15.0154, 35.2553) projected
  line L95 (-15.0154, 35.2553) -> (-15.3379, 34.5779) projected
  circle A45 centre (-46.9705, 30.3822) radius 0.425 projected
  circle A46 centre (-45.9981, 32.7291) radius 0.425 projected
  circle A47 centre (-45.0265, 35.0752) radius 0.425 projected
  circle A48 centre (-43.4319, 38.0486) radius 0.425 projected
  circle A49 centre (-42.0246, 40.1628) radius 0.425 projected
  circle A50 centre (-40.616, 42.277) radius 0.425 projected
  circle A51 centre (-34.8776, 48.4717) radius 0.425 projected
  circle A52 centre (-38.4755, 44.8854) radius 0.425 projected
  circle A53 centre (-36.6766, 46.6786) radius 0.425 projected
  circle A54 centre (28.0325, -9.7061) radius 0.425 projected
  circle A55 centre (29.4807, -7.6188) radius 0.425 projected
  circle A56 centre (30.9282, -5.5321) radius 0.425 projected
  circle A57 centre (32.4825, -2.5312) radius 0.425 projected
  circle A58 centre (33.4542, -0.1851) radius 0.425 projected
  circle A59 centre (34.4265, 2.1618) radius 0.425 projected
  circle A60 centre (35.406, 5.3911) radius 0.425 projected
  ellipse E3 centre (26.3253, 5.0294) end of major axis (25.2293, 6.1254) minor radius 1.55 projected
  circle A61 centre (35.9017, 7.8822) radius 0.425 projected
  circle A62 centre (36.3968, 10.3726) radius 0.425 projected
  circle A63 centre (36.7285, 13.7307) radius 0.425 projected
  circle A64 centre (9.8791, 38.23) radius 0.45 projected
  circle A65 centre (36.7286, 16.2706) radius 0.425 projected
  circle A66 centre (36.7287, 18.8105) radius 0.425 projected
  circle A67 centre (36.3972, 22.1686) radius 0.425 projected
  circle A68 centre (35.9023, 24.659) radius 0.425 projected
  circle A69 centre (35.4067, 27.1502) radius 0.425 projected
  circle A70 centre (34.4274, 30.3796) radius 0.425 projected
  circle A71 centre (33.4552, 32.7265) radius 0.425 projected
  circle A72 centre (32.4837, 35.0727) radius 0.425 projected
  circle A73 centre (30.8928, 38.0483) radius 0.425 projected
  circle A74 centre (29.4822, 40.1604) radius 0.425 projected
  circle A75 centre (19.7302, 50.6132) radius 0.425 projected
  circle A76 centre (28.0709, 42.2719) radius 0.425 projected
  circle A77 centre (25.9306, 44.8805) radius 0.425 projected
  circle A78 centre (22.3386, 48.4727) radius 0.425 projected
  circle A79 centre (24.1346, 46.6766) radius 0.425 projected
  circle A80 centre (-4.8414, 42.1747) radius 0.45 projected
  ellipse E4 centre (-17.5153, 48.87) end of major axis (-18.6113, 49.966) minor radius 1.55 projected
  circle A81 centre (-7.295, 42.8324) radius 0.45 projected
  circle A82 centre (0.0652, 40.86) radius 0.45 projected
  circle A83 centre (2.5188, 40.2023) radius 0.45 projected
  circle A84 centre (-2.3884, 41.5177) radius 0.45 projected
  circle A85 centre (-14.659, 58.4462) radius 0.425 projected
  circle A86 centre (-28.0546, 53.446) radius 0.425 projected
  circle A87 centre (-32.2655, 50.6057) radius 0.425 projected
  circle A88 centre (-30.1604, 52.0262) radius 0.425 projected
  circle A89 centre (-20.3796, 56.9714) radius 0.425 projected
  circle A90 centre (-17.1502, 57.9506) radius 0.425 projected
  circle A91 centre (-25.0727, 55.0277) radius 0.425 projected
  circle A92 centre (-22.7265, 55.9992) radius 0.425 projected
  circle A93 centre (7.4254, 38.8877) radius 0.45 projected
  circle A94 centre (4.9725, 39.5446) radius 0.45 projected
  circle A95 centre (7.8382, 56.9705) radius 0.425 projected
  circle A96 centre (15.5067, 53.4354) radius 0.425 projected
  circle A97 centre (17.6188, 52.0247) radius 0.425 projected
  circle A98 centre (10.1851, 55.9981) radius 0.425 projected
  circle A99 centre (12.5312, 55.0265) radius 0.425 projected
  circle A100 centre (-6.2706, 59.2726) radius 0.425 projected
  circle A101 centre (-12.1686, 58.9411) radius 0.425 projected
  circle A102 centre (-8.8105, 59.2727) radius 0.425 projected
  circle A103 centre (2.1178, 58.4457) radius 0.425 projected
  circle A104 centre (4.6089, 57.9499) radius 0.425 projected
  circle A105 centre (-3.7307, 59.2725) radius 0.425 projected
  circle A106 centre (-0.3726, 58.9407) radius 0.425 projected
  circle A107 centre (9.8791, 38.23) radius 0.45
  circle A108 centre (7.4254, 38.8877) radius 0.45
  circle A109 centre (4.9725, 39.5446) radius 0.45
  circle A110 centre (2.5188, 40.2023) radius 0.45
  circle A111 centre (0.0652, 40.86) radius 0.45
  circle A112 centre (-2.3884, 41.5177) radius 0.45
  circle A113 centre (-4.8414, 42.1747) radius 0.45
  circle A114 centre (-7.295, 42.8324) radius 0.45
  circle A115 centre (-5.2489, -10.2884) radius 0.45
  circle A116 centre (-7.7026, -9.6307) radius 0.45
  circle A117 centre (-10.1555, -8.9737) radius 0.45
  circle A118 centre (-12.6092, -8.316) radius 0.45
  circle A119 centre (-15.0628, -7.6583) radius 0.45
  circle A120 centre (-19.9694, -6.3437) radius 0.45
  circle A121 centre (-22.423, -5.686) radius 0.45
  circle A122 centre (-17.5164, -7.0006) radius 0.45
  point P0 (0, 0)
  dimension "d380" = 180
  constraints: 16 centre point, 8 coincident, 8 concentric, 22 other
extrude "Выдавливание15" cut sketch "Эскиз21" against normal blind 10 contours A115 | A116 | A117 | A118 | A119 | A120 | A121 | A122
